Autodesk Fusion 360 part; units mm, degrees
(part 22 of 24)
  line L521 (40.5032, 38.4302) -> (40.7768, 38.4302)
  line L522 (51.1302, 38.2368) -> (51.1302, 37.9632)
  line L523 (50.9368, 37.7698) -> (50.6632, 37.7698)
  line L524 (40.5032, 42.2402) -> (40.7768, 42.2402)
  line L525 (40.7768, 42.2402) -> (40.9702, 42.0468)
  line L526 (50.6632, 42.2402) -> (50.9368, 42.2402)
  line L527 (26.3398, 42.0468) -> (26.5332, 42.2402)
  line L528 (37.1602, 41.7732) -> (36.9668, 41.5798)
  line L529 (50.4698, 38.2368) -> (50.6632, 38.4302)
  line L530 (40.3098, 42.0468) -> (40.5032, 42.2402)
  line L531 (40.9702, 41.7732) -> (40.7768, 41.5798)
  line L532 (51.1302, 42.0468) -> (51.1302, 41.7732)
  line L533 (51.1302, 38.2368) -> (51.1302, 37.9632)
  line L534 (40.5032, 41.5798) -> (40.3098, 41.7732)
  line L535 (50.4698, 41.7732) -> (50.4698, 42.0468)
  line L536 (50.6632, 41.5798) -> (50.4698, 41.7732)
  line L537 (40.7768, 41.5798) -> (40.5032, 41.5798)
  line L538 (50.4698, 41.7732) -> (50.4698, 42.0468)
  line L539 (36.9668, 41.5798) -> (36.6932, 41.5798)
  line L540 (40.3098, 41.7732) -> (40.3098, 42.0468)
  line L541 (26.5332, 41.5798) -> (26.3398, 41.7732)
  line L542 (50.4698, 42.0468) -> (50.6632, 42.2402)
  line L543 (51.1302, 37.9632) -> (50.9368, 37.7698)
  line L544 (50.4698, 41.7732) -> (50.4698, 42.0468)
  line L545 (40.7768, 38.4302) -> (40.9702, 38.2368)
  line L546 (50.4698, 42.0468) -> (50.6632, 42.2402)
  line L547 (50.4698, 41.7732) -> (50.4698, 42.0468)
  line L548 (51.1302, 38.2368) -> (51.1302, 37.9632)
  line L549 (40.9702, 38.2368) -> (40.9702, 37.9632)
  line L550 (40.3098, 41.7732) -> (40.3098, 42.0468)
  line L551 (40.3098, 41.7732) -> (40.3098, 42.0468)
  line L552 (40.5032, 41.5798) -> (40.3098, 41.7732)
  line L553 (50.6632, 41.5798) -> (50.4698, 41.7732)
  line L554 (40.3098, 42.0468) -> (40.5032, 42.2402)
  line L555 (40.3098, 37.9632) -> (40.3098, 38.2368)
  line L556 (50.6632, 42.2402) -> (50.9368, 42.2402)
  line L557 (40.5032, 37.7698) -> (40.3098, 37.9632)
  line L558 (50.9368, 41.5798) -> (50.6632, 41.5798)
  line L559 (40.3098, 38.2368) -> (40.5032, 38.4302)
  line L560 (36.9668, 41.5798) -> (36.6932, 41.5798)
  line L561 (36.4998, 42.0468) -> (36.6932, 42.2402)
  line L562 (4.7498, 15.1032) -> (4.7498, 15.3768)
  line L563 (15.5702, 15.3768) -> (15.5702, 15.1032)
  line L564 (26.8068, 42.2402) -> (27.0002, 42.0468)
  line L565 (5.4102, 15.1032) -> (5.2168, 14.9098)
  line L566 (26.5332, 42.2402) -> (26.8068, 42.2402)
  line L567 (5.2168, 14.9098) -> (4.9432, 14.9098)
  line L568 (26.8068, 42.2402) -> (27.0002, 42.0468)
  line L569 (26.3398, 41.7732) -> (26.3398, 42.0468)
  line L570 (15.3768, 14.9098) -> (15.1032, 14.9098)
  line L571 (15.5702, 15.3768) -> (15.5702, 15.1032)
  line L572 (15.1032, 15.5702) -> (15.3768, 15.5702)
  line L573 (15.3768, 15.5702) -> (15.5702, 15.3768)
  line L574 (26.5332, 42.2402) -> (26.8068, 42.2402)
  line L575 (15.1032, 14.9098) -> (14.9098, 15.1032)
  line L576 (15.3768, 14.9098) -> (15.1032, 14.9098)
  line L577 (4.9432, 15.5702) -> (5.2168, 15.5702)
  line L578 (14.9098, 15.3768) -> (15.1032, 15.5702)
  line L579 (14.9098, 15.3768) -> (15.1032, 15.5702)
  line L580 (15.3768, 15.5702) -> (15.5702, 15.3768)
  line L581 (15.5702, 15.3768) -> (15.5702, 15.1032)
  line L582 (5.4102, 15.3768) -> (5.4102, 15.1032)
  line L583 (5.2168, 14.9098) -> (4.9432, 14.9098)
  line L584 (4.9432, 14.9098) -> (4.7498, 15.1032)
  line L585 (5.2168, 15.5702) -> (5.4102, 15.3768)
  line L586 (5.4102, 15.3768) -> (5.4102, 15.1032)
  line L587 (36.6932, 42.2402) -> (36.9668, 42.2402)
  line L588 (4.7498, 15.3768) -> (4.9432, 15.5702)
  line L589 (27.0002, 41.7732) -> (26.8068, 41.5798)
  line L590 (26.3398, 41.7732) -> (26.3398, 42.0468)
  line L591 (5.4102, 15.3768) -> (5.4102, 15.1032)
  line L592 (4.7498, 15.1032) -> (4.7498, 15.3768)
  line L593 (15.5702, 15.1032) -> (15.3768, 14.9098)
  line L594 (27.0002, 42.0468) -> (27.0002, 41.7732)
  line L595 (36.4998, 42.0468) -> (36.6932, 42.2402)
  line L596 (15.1032, 15.5702) -> (15.3768, 15.5702)
  line L597 (14.9098, 15.1032) -> (14.9098, 15.3768)
  line L598 (37.1602, 42.0468) -> (37.1602, 41.7732)
  line L599 (15.5702, 15.1032) -> (15.3768, 14.9098)
  line L600 (26.3398, 41.7732) -> (26.3398, 42.0468)
  line L601 (26.8068, 41.5798) -> (26.5332, 41.5798)
  line L602 (36.4998, 41.7732) -> (36.4998, 42.0468)
  line L603 (4.7498, 15.3768) -> (4.9432, 15.5702)
  line L604 (5.4102, 15.1032) -> (5.2168, 14.9098)
  line L605 (26.8068, 41.5798) -> (26.5332, 41.5798)
  line L606 (36.4998, 41.7732) -> (36.4998, 42.0468)
  line L607 (27.0002, 41.7732) -> (26.8068, 41.5798)
  line L608 (26.3398, 41.7732) -> (26.3398, 42.0468)
  line L609 (36.6932, 41.5798) -> (36.4998, 41.7732)
  line L610 (36.6932, 42.2402) -> (36.9668, 42.2402)
  line L611 (36.9668, 42.2402) -> (37.1602, 42.0468)
  line L612 (36.6932, 41.5798) -> (36.4998, 41.7732)
  line L613 (27.0002, 42.0468) -> (27.0002, 41.7732)
  line L614 (37.1602, 42.0468) -> (37.1602, 41.7732)
  line L615 (15.5702, 15.3768) -> (15.5702, 15.1032)
  line L616 (14.9098, 15.1032) -> (14.9098, 15.3768)
  line L617 (5.2168, 15.5702) -> (5.4102, 15.3768)
  line L618 (36.9668, 42.2402) -> (37.1602, 42.0468)
  line L619 (37.1602, 41.7732) -> (36.9668, 41.5798)
  line L620 (26.3398, 42.0468) -> (26.5332, 42.2402)
  line L621 (26.5332, 41.5798) -> (26.3398, 41.7732)
  line L622 (15.1032, 14.9098) -> (14.9098, 15.1032)
  line L623 (4.9432, 14.9098) -> (4.7498, 15.1032)
  arc A308 (74.2188, 21.7805) -> (74.2188, 20.8407) centre (74.2188, 21.3106) ccw
  arc A309 (80.7491, 6.9342) -> (80.7491, 7.874) centre (80.7491, 7.4041) ccw
  arc A310 (74.2188, 16.3195) -> (74.2188, 17.2593) centre (74.2188, 16.7894) ccw
  arc A311 (80.7491, 7.874) -> (80.7491, 6.9342) centre (80.7491, 7.4041) ccw
  line L624 (7.8831, 28.575) -> (7.3569, 28.575)
  line L625 (7.8831, 29.845) -> (8.255, 29.4731)
  line L626 (8.255, 29.4731) -> (8.255, 28.9469)
  arc A312 (80.7491, 7.874) -> (80.7491, 6.9342) centre (80.7491, 7.4041) ccw
  arc A313 (80.7212, 17.2593) -> (80.7212, 16.3195) centre (80.7212, 16.7894) ccw
  line L627 (6.985, 28.9469) -> (6.985, 29.4731)
  line L628 (7.3569, 29.845) -> (7.8831, 29.845)
  line L629 (6.985, 21.3269) -> (6.985, 21.8531)
  arc A314 (80.7491, 2.413) -> (80.7491, 3.3528) centre (80.7491, 2.8829) ccw
  line L630 (7.3569, 28.575) -> (6.985, 28.9469)
  arc A315 (80.7212, 16.3195) -> (80.7212, 17.2593) centre (80.7212, 16.7894) ccw
  line L631 (6.985, 28.9469) -> (6.985, 29.4731)
  line L632 (8.255, 21.8531) -> (8.255, 21.3269)
  arc A316 (74.2467, 6.9342) -> (74.2467, 7.874) centre (74.2467, 7.4041) ccw
  arc A317 (80.7212, 20.8407) -> (80.7212, 21.7805) centre (80.7212, 21.3106) ccw
  arc A318 (74.2467, 2.413) -> (74.2467, 3.3528) centre (74.2467, 2.8829) ccw
  arc A319 (74.2188, 20.8407) -> (74.2188, 21.7805) centre (74.2188, 21.3106) ccw
  arc A320 (80.7491, 3.3528) -> (80.7491, 2.413) centre (80.7491, 2.8829) ccw
  arc A321 (80.7212, 20.8407) -> (80.7212, 21.7805) centre (80.7212, 21.3106) ccw
  arc A322 (74.2188, 20.8407) -> (74.2188, 21.7805) centre (74.2188, 21.3106) ccw
  arc A323 (74.2188, 17.2593) -> (74.2188, 16.3195) centre (74.2188, 16.7894) ccw
  arc A324 (74.2188, 17.2593) -> (74.2188, 16.3195) centre (74.2188, 16.7894) ccw
  arc A325 (80.7212, 17.2593) -> (80.7212, 16.3195) centre (80.7212, 16.7894) ccw
  line L633 (4.9432, 15.5702) -> (5.2168, 15.5702)
  arc A326 (74.2467, 7.874) -> (74.2467, 6.9342) centre (74.2467, 7.4041) ccw
  arc A327 (74.2467, 6.9342) -> (74.2467, 7.874) centre (74.2467, 7.4041) ccw
  arc A328 (80.7491, 6.9342) -> (80.7491, 7.874) centre (80.7491, 7.4041) ccw
  arc A329 (80.7212, 21.7805) -> (80.7212, 20.8407) centre (80.7212, 21.3106) ccw
  line L634 (7.8831, 29.845) -> (8.255, 29.4731)
  arc A330 (80.7491, 3.3528) -> (80.7491, 2.413) centre (80.7491, 2.8829) ccw
  arc A331 (80.7212, 21.7805) -> (80.7212, 20.8407) centre (80.7212, 21.3106) ccw
  line L635 (8.255, 29.4731) -> (8.255, 28.9469)
  line L636 (8.255, 28.9469) -> (7.8831, 28.575)
  line L637 (7.8831, 28.575) -> (7.3569, 28.575)
  line L638 (8.255, 28.9469) -> (7.8831, 28.575)
  line L639 (7.3569, 29.845) -> (7.8831, 29.845)
  line L640 (8.255, 21.3269) -> (7.8831, 20.955)
  line L641 (5.4102, 15.3768) -> (5.4102, 15.1032)
  arc A332 (74.2188, 16.3195) -> (74.2188, 17.2593) centre (74.2188, 16.7894) ccw
  line L642 (7.8831, 28.575) -> (7.3569, 28.575)
  line L643 (6.985, 21.8531) -> (7.3569, 22.225)
  arc A333 (80.7491, 2.413) -> (80.7491, 3.3528) centre (80.7491, 2.8829) ccw
  arc A334 (74.2467, 2.413) -> (74.2467, 3.3528) centre (74.2467, 2.8829) ccw
  line L644 (7.8831, 20.955) -> (7.3569, 20.955)
  line L645 (7.8831, 22.225) -> (8.255, 21.8531)
  line L646 (7.8831, 28.575) -> (7.3569, 28.575)
  line L647 (8.255, 21.8531) -> (8.255, 21.3269)
  arc A335 (74.2467, 7.874) -> (74.2467, 6.9342) centre (74.2467, 7.4041) ccw
  line L648 (6.985, 29.4731) -> (7.3569, 29.845)
  line L649 (8.255, 21.3269) -> (7.8831, 20.955)
  line L650 (7.3569, 20.955) -> (6.985, 21.3269)
  line L651 (7.3569, 28.575) -> (6.985, 28.9469)
  arc A336 (74.2467, 3.3528) -> (74.2467, 2.413) centre (74.2467, 2.8829) ccw
  arc A337 (80.7212, 16.3195) -> (80.7212, 17.2593) centre (80.7212, 16.7894) ccw
  arc A338 (74.2188, 21.7805) -> (74.2188, 20.8407) centre (74.2188, 21.3106) ccw
  line L652 (6.985, 29.4731) -> (7.3569, 29.845)
  arc A339 (74.2467, 3.3528) -> (74.2467, 2.413) centre (74.2467, 2.8829) ccw
  line L653 (7.8831, 20.955) -> (7.3569, 20.955)
  line L654 (6.985, 21.3269) -> (6.985, 21.8531)
  line L655 (7.3569, 22.225) -> (7.8831, 22.225)
  arc A340 (20.9804, 37.7698) -> (20.9804, 38.4302) centre (20.9804, 38.1) ccw
  line L656 (7.8831, 20.955) -> (7.3569, 20.955)
  arc A341 (20.9804, 37.7698) -> (20.9804, 38.4302) centre (20.9804, 38.1) ccw
  line L657 (20.9804, 38.1) -> (19.6596, 38.1)
  line L658 (20.9804, 40.64) -> (19.6596, 40.64)
  arc A342 (19.6596, 43.5102) -> (19.6596, 42.8498) centre (19.6596, 43.18) ccw
  line L659 (7.3569, 20.955) -> (6.985, 21.3269)
  arc A343 (20.9804, 40.3098) -> (20.9804, 40.9702) centre (20.9804, 40.64) ccw
  line L660 (20.9804, 43.18) -> (19.6596, 43.18)
  arc A344 (20.9804, 42.8498) -> (20.9804, 43.5102) centre (20.9804, 43.18) ccw
  arc A345 (20.9804, 40.3098) -> (20.9804, 40.9702) centre (20.9804, 40.64) ccw
  line L661 (7.8831, 20.955) -> (7.3569, 20.955)
  arc A346 (19.6596, 43.5102) -> (19.6596, 42.8498) centre (19.6596, 43.18) ccw
  line L662 (20.9804, 38.1) -> (19.6596, 38.1)
  arc A347 (19.6596, 38.4302) -> (19.6596, 37.7698) centre (19.6596, 38.1) ccw
  arc A348 (19.6596, 38.4302) -> (19.6596, 37.7698) centre (19.6596, 38.1) ccw
  line L663 (7.8831, 22.225) -> (8.255, 21.8531)
  arc A349 (19.6596, 40.9702) -> (19.6596, 40.3098) centre (19.6596, 40.64) ccw
  arc A350 (19.6596, 40.9702) -> (19.6596, 40.3098) centre (19.6596, 40.64) ccw
  line L664 (7.3569, 22.225) -> (7.8831, 22.225)
  line L665 (6.985, 21.8531) -> (7.3569, 22.225)
  line L666 (20.9804, 40.64) -> (19.6596, 40.64)
  arc A351 (20.9804, 42.8498) -> (20.9804, 43.5102) centre (20.9804, 43.18) ccw
  line L667 (20.9804, 43.18) -> (19.6596, 43.18)
  line L668 (10.9601, 50.4698) -> (10.9601, 48.5902)
  line L669 (11.8999, 48.5902) -> (11.8999, 50.4698)
  line L670 (13.5001, 50.4698) -> (13.5001, 48.5902)
  line L671 (14.4399, 48.5902) -> (14.4399, 50.4698)
  line L672 (16.0401, 50.4698) -> (16.0401, 48.5902)
  line L673 (16.9799, 50.4698) -> (16.9799, 48.5902)
  line L674 (18.5801, 48.5902) -> (18.5801, 50.4698)
  line L675 (19.5199, 50.4698) -> (19.5199, 48.5902)
  line L676 (21.1201, 48.5902) -> (21.1201, 50.4698)
  line L677 (22.0599, 50.4698) -> (22.0599, 48.5902)
  line L678 (20.9804, 43.5102) -> (19.6596, 43.5102)
  line L679 (19.6596, 42.8498) -> (20.9804, 42.8498)
  line L680 (20.9804, 40.9702) -> (19.6596, 40.9702)
  line L681 (19.6596, 40.3098) -> (20.9804, 40.3098)
  line L682 (20.9804, 38.4302) -> (19.6596, 38.4302)
  line L683 (19.6596, 37.7698) -> (20.9804, 37.7698)
  line L684 (3.7084, 44.7802) -> (2.3876, 44.7802)
  line L685 (2.3876, 44.1198) -> (3.7084, 44.1198)
  line L686 (7.4676, 44.7802) -> (8.7884, 44.7802)
  line L687 (8.7884, 44.1198) -> (7.4676, 44.1198)
  line L688 (7.4676, 42.2402) -> (8.7884, 42.2402)
  line L689 (8.7884, 41.5798) -> (7.4676, 41.5798)
  line L690 (3.7084, 42.2402) -> (2.3876, 42.2402)
  line L691 (2.3876, 41.5798) -> (3.7084, 41.5798)
  line L692 (2.3876, 34.6202) -> (3.7084, 34.6202)
  line L693 (3.7084, 33.9598) -> (2.3876, 33.9598)
  line L694 (8.7884, 34.6202) -> (7.4676, 34.6202)
  line L695 (7.4676, 33.9598) -> (8.7884, 33.9598)
  line L696 (26.2001, 26.3398) -> (26.2001, 24.4602)
  line L697 (27.1399, 26.3398) -> (27.1399, 24.4602)
  line L698 (28.7401, 26.3398) -> (28.7401, 24.4602)
  line L699 (29.6799, 26.3398) -> (29.6799, 24.4602)
  line L700 (31.2801, 24.4602) -> (31.2801, 26.3398)
  line L701 (32.2199, 26.3398) -> (32.2199, 24.4602)
  line L702 (33.8201, 24.4602) -> (33.8201, 26.3398)
  line L703 (34.7599, 26.3398) -> (34.7599, 24.4602)
  line L704 (36.3601, 24.4602) -> (36.3601, 26.3398)
  line L705 (37.2999, 26.3398) -> (37.2999, 24.4602)
  line L706 (47.7901, 26.3398) -> (47.7901, 24.4602)
  line L707 (48.7299, 24.4602) -> (48.7299, 26.3398)
  line L708 (50.3301, 26.3398) -> (50.3301, 24.4602)
  line L709 (51.2699, 24.4602) -> (51.2699, 26.3398)
  line L710 (52.8701, 26.3398) -> (52.8701, 24.4602)
  line L711 (53.8099, 24.4602) -> (53.8099, 26.3398)
  line L712 (60.4901, 30.8102) -> (60.4901, 32.6898)
  line L713 (61.4299, 30.8102) -> (61.4299, 32.6898)
  line L714 (63.0301, 32.6898) -> (63.0301, 30.8102)
  line L715 (63.9699, 30.8102) -> (63.9699, 32.6898)
  line L716 (65.5701, 32.6898) -> (65.5701, 30.8102)
  line L717 (66.5099, 30.8102) -> (66.5099, 32.6898)
  line L718 (73.1901, 32.6898) -> (73.1901, 30.8102)
  line L719 (74.1299, 30.8102) -> (74.1299, 32.6898)
  line L720 (75.7301, 32.6898) -> (75.7301, 30.8102)
  line L721 (76.6699, 30.8102) -> (76.6699, 32.6898)
  line L722 (78.2701, 32.6898) -> (78.2701, 30.8102)
  line L723 (79.2099, 30.8102) -> (79.2099, 32.6898)
  line L724 (80.8101, 32.6898) -> (80.8101, 30.8102)
  line L725 (81.7499, 30.8102) -> (81.7499, 32.6898)
  line L726 (57.9501, 44.1198) -> (57.9501, 42.2402)
  line L727 (58.8899, 42.2402) -> (58.8899, 44.1198)
  line L728 (60.4901, 44.1198) -> (60.4901, 42.2402)
  line L729 (61.4299, 42.2402) -> (61.4299, 44.1198)
  line L730 (63.0301, 44.1198) -> (63.0301, 42.2402)
  line L731 (63.9699, 42.2402) -> (63.9699, 44.1198)
  line L732 (65.5701, 44.1198) -> (65.5701, 42.2402)
  line L733 (66.5099, 42.2402) -> (66.5099, 44.1198)
  line L734 (73.1901, 45.3898) -> (73.1901, 43.5102)
  line L735 (74.1299, 43.5102) -> (74.1299, 45.3898)
  line L736 (75.7301, 45.3898) -> (75.7301, 43.5102)
  line L737 (76.6699, 43.5102) -> (76.6699, 45.3898)
  line L738 (79.2099, 45.3898) -> (79.2099, 43.5102)
  line L739 (78.2701, 43.5102) -> (78.2701, 45.3898)
  line L740 (80.8101, 45.3898) -> (80.8101, 43.5102)
  line L741 (81.7499, 43.5102) -> (81.7499, 45.3898)
  constraint tangent A238 L668
  constraint tangent A222 L669
  constraint tangent A226 L670
  constraint tangent A221 L671
  constraint tangent A236 L672
  constraint tangent A231 L673
  constraint tangent A217 L674
  constraint tangent A225 L675
  constraint tangent A224 L676
  constraint tangent A237 L677
  constraint tangent A346 L678
  constraint tangent A344 L679
  constraint tangent A349 L680
  constraint tangent A350 L681
  constraint parallel L680 L681
  constraint tangent A347 L682
  constraint tangent A341 L683
  constraint tangent A280 L684
  constraint tangent A283 L685
  constraint tangent A292 L686
  constraint tangent A297 L687
  constraint tangent A295 L688
  constraint tangent A289 L689
  constraint tangent A296 L690
  constraint tangent A288 L691
  constraint tangent A303 L692
  constraint tangent A301 L693
  constraint tangent A293 L694
  constraint tangent A286 L695
  constraint tangent A153 L696
  constraint tangent A100 L697
  constraint tangent A136 L698
  constraint tangent A136 L699
  constraint tangent A151 L700
  constraint tangent A154 L701
  constraint tangent A152 L702
  constraint tangent A152 L703
  constraint tangent A149 L704
  constraint tangent A147 L705
  constraint tangent A252 L706
  constraint tangent A264 L707
  constraint tangent A257 L708
  constraint tangent A249 L709
  constraint tangent A268 L710
  constraint tangent A266 L711
  constraint tangent A213 L712
  constraint tangent A213 L713
  constraint tangent A198 L714
  constraint tangent A229 L715
  constraint tangent A218 L716
  constraint tangent A218 L717
  constraint tangent A163 L718
  constraint tangent A180 L719
  constraint tangent A168 L720
  constraint tangent A170 L721
  constraint tangent A208 L722
  constraint tangent A208 L723
  constraint tangent A206 L724
  constraint tangent A186 L725
  constraint tangent A209 L726
  constraint tangent A209 L727
  constraint tangent A187 L728
  constraint tangent A204 L729
  constraint tangent A195 L730
  constraint tangent A194 L731
  constraint tangent A185 L732
  constraint tangent A191 L733
  constraint tangent A160 L734
  constraint tangent A169 L735
  constraint tangent A176 L736
  constraint tangent A166 L737
  constraint tangent A181 L738
  constraint tangent A159 L739
  constraint tangent A162 L740
  constraint tangent A158 L741
sketch "Bottom Component Outlines" plane through (0, 0, 0) normal (0, 0, 1) x (1, 0, 0)
  arc A0 (46.3191, 48.2959) -> (46.3909, 48.2241) centre (46.355, 48.26) ccw
  line L0 (59.055, 7.62) -> (57.785, 7.62)
  arc A1 (67.9809, 7.5841) -> (67.9091, 7.6559) centre (67.945, 7.62) ccw
  arc A2 (67.2741, 7.0209) -> (67.3459, 6.9491) centre (67.31, 6.985) ccw
  arc A3 (52.705, 7.6708) -> (52.705, 7.5692) centre (52.705, 7.62) ccw
  arc A4 (53.9391, 5.1159) -> (54.0109, 5.0441) centre (53.975, 5.08) ccw
  arc A5 (51.3991, 5.1159) -> (51.4709, 5.0441) centre (51.435, 5.08) ccw
  arc A6 (49.4941, 7.0209) -> (49.5659, 6.9491) centre (49.53, 6.985) ccw
  arc A7 (69.215, 7.5692) -> (69.215, 7.6708) centre (69.215, 7.62) ccw
  arc A8 (49.5659, 5.7509) -> (49.4941, 5.6791) centre (49.53, 5.715) ccw
  arc A9 (52.705, 5.1308) -> (52.705, 5.0292) centre (52.705, 5.08) ccw
  arc A10 (67.9091, 5.0441) -> (67.9809, 5.1159) centre (67.945, 5.08) ccw
  arc A11 (54.5741, 6.9491) -> (54.6459, 7.0209) centre (54.61, 6.985) ccw
  line L1 (52.07, 6.985) -> (51.435, 7.62)
  line L2 (54.61, 6.985) -> (53.975, 7.62)
  line L3 (52.07, 5.715) -> (52.705, 5.08)
  line L4 (51.435, 5.08) -> (52.07, 5.715)
  arc A12 (52.7409, 7.5841) -> (52.6691, 7.6559) centre (52.705, 7.62) ccw
  arc A13 (50.1291, 5.0441) -> (50.2009, 5.1159) centre (50.165, 5.08) ccw
  arc A14 (54.6459, 5.6791) -> (54.5741, 5.7509) centre (54.61, 5.715) ccw
  arc A15 (69.7992, 5.715) -> (69.9008, 5.715) centre (69.85, 5.715) ccw
  arc A16 (51.4709, 7.6559) -> (51.3991, 7.5841) centre (51.435, 7.62) ccw
  arc A17 (46.3909, 50.8359) -> (46.3191, 50.7641) centre (46.355, 50.8) ccw
  line L5 (69.85, 6.985) -> (69.215, 7.62)
  arc A18 (52.1059, 5.7509) -> (52.0341, 5.6791) centre (52.07, 5.715) ccw
  line L6 (69.85, 5.715) -> (69.85, 6.985)
  arc A19 (69.1791, 5.1159) -> (69.2509, 5.0441) centre (69.215, 5.08) ccw
  arc A20 (54.0109, 7.6559) -> (53.9391, 7.5841) centre (53.975, 7.62) ccw
  line L7 (52.705, 5.08) -> (53.975, 5.08)
  arc A21 (52.0341, 7.0209) -> (52.1059, 6.9491) centre (52.07, 6.985) ccw
  arc A22 (69.2509, 7.6559) -> (69.1791, 7.5841) centre (69.215, 7.62) ccw
  line L8 (45.085, 48.26) -> (46.355, 48.26)
  arc A23 (52.705, 50.8508) -> (52.705, 50.7492) centre (52.705, 50.8) ccw
  arc A24 (69.9008, 6.985) -> (69.7992, 6.985) centre (69.85, 6.985) ccw
  line L9 (67.31, 6.985) -> (67.945, 7.62)
  arc A25 (53.975, 7.5692) -> (53.975, 7.6708) centre (53.975, 7.62) ccw
  line L10 (52.705, 7.62) -> (52.07, 6.985)
  arc A26 (52.1059, 5.6791) -> (52.0341, 5.7509) centre (52.07, 5.715) ccw
  arc A27 (52.6691, 5.0441) -> (52.7409, 5.1159) centre (52.705, 5.08) ccw
  line L11 (53.975, 7.62) -> (52.705, 7.62)
  arc A28 (51.435, 7.5692) -> (51.435, 7.6708) centre (51.435, 7.62) ccw
  arc A29 (67.945, 5.1308) -> (67.945, 5.0292) centre (67.945, 5.08) ccw
  line L12 (69.215, 5.08) -> (69.85, 5.715)
  arc A30 (50.165, 5.1308) -> (50.165, 5.0292) centre (50.165, 5.08) ccw
  arc A31 (57.785, 7.6708) -> (57.785, 7.5692) centre (57.785, 7.62) ccw
  arc A32 (47.0259, 48.8591) -> (46.9541, 48.9309) centre (46.99, 48.895) ccw
  arc A33 (59.055, 7.5692) -> (59.055, 7.6708) centre (59.055, 7.62) ccw
  arc A34 (69.215, 5.0292) -> (69.215, 5.1308) centre (69.215, 5.08) ccw
  arc A35 (51.435, 5.0292) -> (51.435, 5.1308) centre (51.435, 5.08) ccw
  line L13 (53.975, 5.08) -> (54.61, 5.715)
  line L14 (51.435, 7.62) -> (50.165, 7.62)
  line L15 (50.165, 5.08) -> (49.53, 5.715)
  line L16 (69.215, 7.62) -> (67.945, 7.62)
  arc A36 (67.945, 7.6708) -> (67.945, 7.5692) centre (67.945, 7.62) ccw
  line L17 (67.945, 5.08) -> (67.31, 5.715)
  arc A37 (50.2009, 7.5841) -> (50.1291, 7.6559) centre (50.165, 7.62) ccw
  arc A38 (50.165, 7.6708) -> (50.165, 7.5692) centre (50.165, 7.62) ccw
  line L18 (52.07, 48.895) -> (52.705, 48.26)
  arc A39 (52.0341, 6.9491) -> (52.1059, 7.0209) centre (52.07, 6.985) ccw
  line L19 (67.945, 5.08) -> (69.215, 5.08)
  line L20 (50.165, 5.08) -> (51.435, 5.08)
  line L21 (49.53, 6.985) -> (50.165, 7.62)
  arc A40 (67.3459, 5.7509) -> (67.2741, 5.6791) centre (67.31, 5.715) ccw
  arc A41 (69.8859, 5.6791) -> (69.8141, 5.7509) centre (69.85, 5.715) ccw
  arc A42 (52.0341, 50.2009) -> (52.1059, 50.1291) centre (52.07, 50.165) ccw
  arc A43 (46.9541, 50.2009) -> (47.0259, 50.1291) centre (46.99, 50.165) ccw
  line L22 (53.975, 50.8) -> (52.705, 50.8)
  arc A44 (46.355, 48.2092) -> (46.355, 48.3108) centre (46.355, 48.26) ccw
  arc A45 (45.0491, 48.2241) -> (45.1209, 48.2959) centre (45.085, 48.26) ccw
  arc A46 (48.895, 50.7492) -> (48.895, 50.8508) centre (48.895, 50.8) ccw
  arc A47 (45.085, 48.3108) -> (45.085, 48.2092) centre (45.085, 48.26) ccw
  line L23 (48.895, 50.8) -> (47.625, 50.8)
  line L24 (46.355, 50.8) -> (45.085, 50.8)
  line L25 (47.625, 50.8) -> (46.99, 50.165)
  arc A48 (49.4941, 50.1291) -> (49.5659, 50.2009) centre (49.53, 50.165) ccw
  line L26 (44.45, 48.895) -> (45.085, 48.26)
  arc A49 (49.5659, 48.8591) -> (49.4941, 48.9309) centre (49.53, 48.895) ccw
  arc A50 (46.9541, 50.1291) -> (47.0259, 50.2009) centre (46.99, 50.165) ccw
  arc A51 (44.4859, 48.9309) -> (44.4141, 48.8591) centre (44.45, 48.895) ccw
  arc A52 (45.1209, 50.7641) -> (45.0491, 50.8359) centre (45.085, 50.8) ccw
  arc A53 (50.2009, 50.7641) -> (50.1291, 50.8359) centre (50.165, 50.8) ccw
  arc A54 (44.4141, 50.2009) -> (44.4859, 50.1291) centre (44.45, 50.165) ccw
  line L27 (49.53, 50.165) -> (48.895, 50.8)
  line L28 (47.625, 48.26) -> (48.895, 48.26)
  line L29 (55.245, 48.26) -> (56.515, 48.26)
  arc A55 (47.0259, 48.9309) -> (46.9541, 48.8591) centre (46.99, 48.895) ccw
  line L30 (52.07, 50.165) -> (51.435, 50.8)
  line L31 (45.085, 50.8) -> (44.45, 50.165)
  arc A56 (52.7409, 50.7641) -> (52.6691, 50.8359) centre (52.705, 50.8) ccw
  arc A57 (47.6609, 50.7641) -> (47.5891, 50.8359) centre (47.625, 50.8) ccw
  arc A58 (46.355, 50.7492) -> (46.355, 50.8508) centre (46.355, 50.8) ccw
  line L32 (49.53, 48.895) -> (50.165, 48.26)
  arc A59 (55.2091, 48.2241) -> (55.2809, 48.2959) centre (55.245, 48.26) ccw
  arc A60 (47.5891, 48.2241) -> (47.6609, 48.2959) centre (47.625, 48.26) ccw
  line L33 (46.99, 48.895) -> (46.355, 48.26)
  line L34 (56.515, 50.8) -> (55.245, 50.8)
  arc A61 (53.975, 48.2092) -> (53.975, 48.3108) centre (53.975, 48.26) ccw
  arc A62 (48.8591, 48.2959) -> (48.9309, 48.2241) centre (48.895, 48.26) ccw
  arc A63 (48.895, 48.2092) -> (48.895, 48.3108) centre (48.895, 48.26) ccw
  line L35 (52.705, 50.8) -> (52.07, 50.165)
  arc A64 (47.625, 50.8508) -> (47.625, 50.7492) centre (47.625, 50.8) ccw
  arc A65 (48.9309, 50.8359) -> (48.8591, 50.7641) centre (48.895, 50.8) ccw
  arc A66 (53.975, 50.7492) -> (53.975, 50.8508) centre (53.975, 50.8) ccw
  arc A67 (45.085, 50.8508) -> (45.085, 50.7492) centre (45.085, 50.8) ccw
  arc A68 (47.625, 48.3108) -> (47.625, 48.2092) centre (47.625, 48.26) ccw
  line L36 (46.99, 48.895) -> (47.625, 48.26)
  line L37 (48.895, 48.26) -> (49.53, 48.895)
  line L38 (46.355, 50.8) -> (46.99, 50.165)
  arc A69 (59.055, 50.7492) -> (59.055, 50.8508) centre (59.055, 50.8) ccw
  arc A70 (51.435, 50.7492) -> (51.435, 50.8508) centre (51.435, 50.8) ccw
  arc A71 (50.165, 50.8508) -> (50.165, 50.7492) centre (50.165, 50.8) ccw
  arc A72 (56.515, 50.7492) -> (56.515, 50.8508) centre (56.515, 50.8) ccw
  line L39 (59.055, 50.8) -> (57.785, 50.8)
  line L40 (50.165, 50.8) -> (49.53, 50.165)
  arc A73 (59.6541, 50.1291) -> (59.7259, 50.2009) centre (59.69, 50.165) ccw
  arc A74 (61.595, 50.7492) -> (61.595, 50.8508) centre (61.595, 50.8) ccw
  arc A75 (52.1059, 48.9309) -> (52.0341, 48.8591) centre (52.07, 48.895) ccw
  line L41 (54.61, 48.895) -> (55.245, 48.26)
  arc A76 (54.6459, 48.8591) -> (54.5741, 48.9309) centre (54.61, 48.895) ccw
  arc A77 (55.245, 50.8508) -> (55.245, 50.7492) centre (55.245, 50.8) ccw
  arc A78 (60.2891, 48.2241) -> (60.3609, 48.2959) centre (60.325, 48.26) ccw
  arc A79 (52.6691, 48.2241) -> (52.7409, 48.2959) centre (52.705, 48.26) ccw
  arc A80 (60.3609, 50.7641) -> (60.2891, 50.8359) centre (60.325, 50.8) ccw
  arc A81 (52.0341, 50.1291) -> (52.1059, 50.2009) centre (52.07, 50.165) ccw
  arc A82 (51.4709, 50.8359) -> (51.3991, 50.7641) centre (51.435, 50.8) ccw
  line L42 (61.595, 50.8) -> (60.325, 50.8)
  line L43 (51.435, 50.8) -> (50.165, 50.8)
  arc A83 (57.1141, 50.1291) -> (57.1859, 50.2009) centre (57.15, 50.165) ccw
  line L44 (57.15, 50.165) -> (56.515, 50.8)
  arc A84 (50.165, 48.3108) -> (50.165, 48.2092) centre (50.165, 48.26) ccw
  arc A85 (55.2809, 50.7641) -> (55.2091, 50.8359) centre (55.245, 50.8) ccw
  line L45 (51.435, 48.26) -> (52.07, 48.895)
  arc A86 (57.1141, 50.2009) -> (57.1859, 50.1291) centre (57.15, 50.165) ccw
  arc A87 (51.435, 48.2092) -> (51.435, 48.3108) centre (51.435, 48.26) ccw
  arc A88 (55.245, 48.3108) -> (55.245, 48.2092) centre (55.245, 48.26) ccw
  arc A89 (52.705, 48.3108) -> (52.705, 48.2092) centre (52.705, 48.26) ccw
  arc A90 (60.325, 50.8508) -> (60.325, 50.7492) centre (60.325, 50.8) ccw
  line L46 (59.69, 48.895) -> (60.325, 48.26)
  arc A91 (49.5659, 48.9309) -> (49.4941, 48.8591) centre (49.53, 48.895) ccw
  line L47 (54.61, 48.895) -> (53.975, 48.26)
  line L48 (50.165, 48.26) -> (51.435, 48.26)
  line L49 (57.785, 50.8) -> (57.15, 50.165)
  arc A92 (56.5509, 50.8359) -> (56.4791, 50.7641) centre (56.515, 50.8) ccw
  arc A93 (54.5741, 50.1291) -> (54.6459, 50.2009) centre (54.61, 50.165) ccw
  arc A94 (49.4941, 50.2009) -> (49.5659, 50.1291) centre (49.53, 50.165) ccw
  arc A95 (53.9391, 48.2959) -> (54.0109, 48.2241) centre (53.975, 48.26) ccw
  arc A96 (52.1059, 48.8591) -> (52.0341, 48.9309) centre (52.07, 48.895) ccw
  line L50 (52.705, 48.26) -> (53.975, 48.26)
  arc A97 (54.6459, 48.9309) -> (54.5741, 48.8591) centre (54.61, 48.895) ccw
  arc A98 (54.5741, 50.2009) -> (54.6459, 50.1291) centre (54.61, 50.165) ccw
  arc A99 (57.785, 50.8508) -> (57.785, 50.7492) centre (57.785, 50.8) ccw
  arc A100 (57.1859, 48.8591) -> (57.1141, 48.9309) centre (57.15, 48.895) ccw
  arc A101 (59.0191, 48.2959) -> (59.0909, 48.2241) centre (59.055, 48.26) ccw
  arc A102 (51.3991, 48.2959) -> (51.4709, 48.2241) centre (51.435, 48.26) ccw
  line L51 (57.785, 48.26) -> (59.055, 48.26)
  line L52 (60.325, 50.8) -> (59.69, 50.165)
  arc A103 (54.0109, 50.8359) -> (53.9391, 50.7641) centre (53.975, 50.8) ccw
  line L53 (56.515, 48.26) -> (57.15, 48.895)
  line L54 (59.69, 50.165) -> (59.055, 50.8)
  arc A104 (59.0909, 50.8359) -> (59.0191, 50.7641) centre (59.055, 50.8) ccw
  line L55 (55.245, 50.8) -> (54.61, 50.165)
  arc A105 (28.575, 50.7492) -> (28.575, 50.8508) centre (28.575, 50.8) ccw
  arc A106 (26.7059, 48.9309) -> (26.6341, 48.8591) centre (26.67, 48.895) ccw
  arc A107 (29.2459, 48.9309) -> (29.1741, 48.8591) centre (29.21, 48.895) ccw
  arc A108 (26.6341, 50.2009) -> (26.7059, 50.1291) centre (26.67, 50.165) ccw
  arc A109 (31.1509, 50.8359) -> (31.0791, 50.7641) centre (31.115, 50.8) ccw
  line L56 (34.925, 50.8) -> (34.29, 50.165)
  arc A110 (56.4791, 48.2959) -> (56.5509, 48.2241) centre (56.515, 48.26) ccw
  line L57 (28.575, 50.8) -> (29.21, 50.165)
  arc A111 (56.515, 48.2092) -> (56.515, 48.3108) centre (56.515, 48.26) ccw
  arc A112 (57.785, 48.3108) -> (57.785, 48.2092) centre (57.785, 48.26) ccw
  arc A113 (62.2659, 48.8591) -> (62.1941, 48.9309) centre (62.23, 48.895) ccw
  line L58 (29.21, 48.895) -> (28.575, 48.26)
  arc A114 (29.1741, 50.2009) -> (29.2459, 50.1291) centre (29.21, 50.165) ccw
  line L59 (59.055, 48.26) -> (59.69, 48.895)
  line L60 (29.845, 48.26) -> (31.115, 48.26)
  arc A115 (50.1291, 48.2241) -> (50.2009, 48.2959) centre (50.165, 48.26) ccw
  arc A116 (62.1941, 50.1291) -> (62.2659, 50.2009) centre (62.23, 50.165) ccw
  arc A117 (62.1792, 48.895) -> (62.2808, 48.895) centre (62.23, 48.895) ccw
  arc A118 (34.9609, 50.7641) -> (34.8891, 50.8359) centre (34.925, 50.8) ccw
  arc A119 (31.115, 48.2092) -> (31.115, 48.3108) centre (31.115, 48.26) ccw
  line L61 (29.845, 50.8) -> (29.21, 50.165)
  line L62 (31.75, 50.165) -> (31.115, 50.8)
  line L63 (27.305, 50.8) -> (26.67, 50.165)
  arc A120 (59.6541, 50.2009) -> (59.7259, 50.1291) centre (59.69, 50.165) ccw
  arc A121 (27.3409, 50.7641) -> (27.2691, 50.8359) centre (27.305, 50.8) ccw
  arc A122 (57.7491, 48.2241) -> (57.8209, 48.2959) centre (57.785, 48.26) ccw
  arc A123 (34.2541, 50.2009) -> (34.3259, 50.1291) centre (34.29, 50.165) ccw
  arc A124 (61.595, 48.2092) -> (61.595, 48.3108) centre (61.595, 48.26) ccw
  arc A125 (31.115, 50.7492) -> (31.115, 50.8508) centre (31.115, 50.8) ccw
  line L64 (53.975, 50.8) -> (54.61, 50.165)
  arc A126 (62.2808, 50.165) -> (62.1792, 50.165) centre (62.23, 50.165) ccw
  arc A127 (59.7259, 48.9309) -> (59.6541, 48.8591) centre (59.69, 48.895) ccw
  arc A128 (34.925, 50.8508) -> (34.925, 50.7492) centre (34.925, 50.8) ccw
  line L65 (62.23, 50.165) -> (62.23, 48.895)
  line L66 (62.23, 48.895) -> (61.595, 48.26)
  arc A129 (59.7259, 48.8591) -> (59.6541, 48.9309) centre (59.69, 48.895) ccw
  arc A130 (36.8659, 48.8591) -> (36.7941, 48.9309) centre (36.83, 48.895) ccw
  arc A131 (37.465, 48.3108) -> (37.465, 48.2092) centre (37.465, 48.26) ccw
  arc A132 (36.8659, 48.9309) -> (36.7941, 48.8591) centre (36.83, 48.895) ccw
  arc A133 (39.4059, 48.8591) -> (39.3341, 48.9309) centre (39.37, 48.895) ccw
  line L67 (57.15, 48.895) -> (57.785, 48.26)
  arc A134 (60.325, 48.3108) -> (60.325, 48.2092) centre (60.325, 48.26) ccw
  arc A135 (29.8809, 50.7641) -> (29.8091, 50.8359) centre (29.845, 50.8) ccw
  arc A136 (29.2459, 48.8591) -> (29.1741, 48.9309) centre (29.21, 48.895) ccw
  line L68 (60.325, 48.26) -> (61.595, 48.26)
  line L69 (29.21, 48.895) -> (29.845, 48.26)
  line L70 (31.115, 48.26) -> (31.75, 48.895)
  arc A137 (29.845, 50.8508) -> (29.845, 50.7492) centre (29.845, 50.8) ccw
  arc A138 (61.5591, 48.2959) -> (61.6309, 48.2241) centre (61.595, 48.26) ccw
  arc A139 (34.3259, 48.8591) -> (34.2541, 48.9309) centre (34.29, 48.895) ccw
  line L71 (34.29, 50.165) -> (33.655, 50.8)
  arc A140 (43.815, 50.7492) -> (43.815, 50.8508) centre (43.815, 50.8) ccw
  arc A141 (57.8209, 50.7641) -> (57.7491, 50.8359) centre (57.785, 50.8) ccw
  line L72 (32.385, 50.8) -> (31.75, 50.165)
  arc A142 (61.6309, 50.8359) -> (61.5591, 50.7641) centre (61.595, 50.8) ccw
  line L73 (27.305, 48.26) -> (28.575, 48.26)
  arc A143 (27.305, 50.8508) -> (27.305, 50.7492) centre (27.305, 50.8) ccw
  line L74 (36.195, 50.8) -> (36.83, 50.165)
  line L75 (31.115, 50.8) -> (29.845, 50.8)
  arc A144 (28.5391, 48.2959) -> (28.6109, 48.2241) centre (28.575, 48.26) ccw
  arc A145 (31.7141, 50.1291) -> (31.7859, 50.2009) centre (31.75, 50.165) ccw
  arc A146 (29.8091, 48.2241) -> (29.8809, 48.2959) centre (29.845, 48.26) ccw
  line L76 (26.67, 48.895) -> (27.305, 48.26)
  arc A147 (57.1859, 48.9309) -> (57.1141, 48.8591) centre (57.15, 48.895) ccw
  arc A148 (31.7859, 48.8591) -> (31.7141, 48.9309) centre (31.75, 48.895) ccw
  arc A149 (34.2541, 50.1291) -> (34.3259, 50.2009) centre (34.29, 50.165) ccw
  line L77 (28.575, 50.8) -> (27.305, 50.8)
  line L78 (36.195, 50.8) -> (34.925, 50.8)
  arc A150 (29.1741, 50.1291) -> (29.2459, 50.2009) centre (29.21, 50.165) ccw
  arc A151 (31.0791, 48.2959) -> (31.1509, 48.2241) centre (31.115, 48.26) ccw
  arc A152 (27.2691, 48.2241) -> (27.3409, 48.2959) centre (27.305, 48.26) ccw
  arc A153 (36.195, 50.7492) -> (36.195, 50.8508) centre (36.195, 50.8) ccw
  line L79 (36.83, 48.895) -> (37.465, 48.26)
  arc A154 (28.6109, 50.8359) -> (28.5391, 50.7641) centre (28.575, 50.8) ccw
  line L80 (33.655, 50.8) -> (32.385, 50.8)
  arc A155 (41.9459, 48.9309) -> (41.8741, 48.8591) centre (41.91, 48.895) ccw
  arc A156 (29.845, 48.3108) -> (29.845, 48.2092) centre (29.845, 48.26) ccw
  arc A157 (59.055, 48.2092) -> (59.055, 48.3108) centre (59.055, 48.26) ccw
  line L81 (61.595, 50.8) -> (62.23, 50.165)
  arc A158 (28.575, 48.2092) -> (28.575, 48.3108) centre (28.575, 48.26) ccw
  arc A159 (27.305, 48.3108) -> (27.305, 48.2092) centre (27.305, 48.26) ccw
  arc A160 (32.385, 48.3108) -> (32.385, 48.2092) centre (32.385, 48.26) ccw
  line L82 (34.29, 48.895) -> (34.925, 48.26)
  arc A161 (42.5809, 50.7641) -> (42.5091, 50.8359) centre (42.545, 50.8) ccw
  line L83 (31.75, 48.895) -> (32.385, 48.26)
  arc A162 (42.545, 50.8508) -> (42.545, 50.7492) centre (42.545, 50.8) ccw
  line L84 (32.385, 48.26) -> (33.655, 48.26)
  line L85 (33.655, 48.26) -> (34.29, 48.895)
  arc A163 (39.3341, 50.1291) -> (39.4059, 50.2009) centre (39.37, 50.165) ccw
  line L86 (41.91, 48.895) -> (42.545, 48.26)
  arc A164 (33.655, 50.7492) -> (33.655, 50.8508) centre (33.655, 50.8) ccw
  arc A165 (42.5091, 48.2241) -> (42.5809, 48.2959) centre (42.545, 48.26) ccw
  arc A166 (41.3109, 50.8359) -> (41.2391, 50.7641) centre (41.275, 50.8) ccw
  line L87 (43.815, 50.8) -> (42.545, 50.8)
  arc A167 (36.2309, 50.8359) -> (36.1591, 50.7641) centre (36.195, 50.8) ccw
  arc A168 (34.8891, 48.2241) -> (34.9609, 48.2959) centre (34.925, 48.26) ccw
  arc A169 (38.7709, 50.8359) -> (38.6991, 50.7641) centre (38.735, 50.8) ccw
  line L88 (38.735, 48.26) -> (39.37, 48.895)
  arc A170 (36.1591, 48.2959) -> (36.2309, 48.2241) centre (36.195, 48.26) ccw
  line L89 (41.91, 50.165) -> (41.275, 50.8)
  arc A171 (32.3491, 48.2241) -> (32.4209, 48.2959) centre (32.385, 48.26) ccw
  arc A172 (33.6909, 50.8359) -> (33.6191, 50.7641) centre (33.655, 50.8) ccw
  line L90 (40.005, 50.8) -> (39.37, 50.165)
  line L91 (36.83, 48.895) -> (36.195, 48.26)
  line L92 (42.545, 50.8) -> (41.91, 50.165)
  arc A173 (33.655, 48.2092) -> (33.655, 48.3108) centre (33.655, 48.26) ccw
  arc A174 (33.6191, 48.2959) -> (33.6909, 48.2241) centre (33.655, 48.26) ccw
  arc A175 (32.4209, 50.7641) -> (32.3491, 50.8359) centre (32.385, 50.8) ccw
  line L93 (37.465, 50.8) -> (36.83, 50.165)
  arc A176 (31.7859, 48.9309) -> (31.7141, 48.8591) centre (31.75, 48.895) ccw
  line L94 (34.925, 48.26) -> (36.195, 48.26)
  arc A177 (36.195, 48.2092) -> (36.195, 48.3108) centre (36.195, 48.26) ccw
  arc A178 (36.7941, 50.1291) -> (36.8659, 50.2009) centre (36.83, 50.165) ccw
  line L95 (38.735, 50.8) -> (37.465, 50.8)
  arc A179 (34.925, 48.3108) -> (34.925, 48.2092) centre (34.925, 48.26) ccw
  arc A180 (37.5009, 50.7641) -> (37.4291, 50.8359) centre (37.465, 50.8) ccw
  arc A181 (31.7141, 50.2009) -> (31.7859, 50.1291) centre (31.75, 50.165) ccw
  arc A182 (38.735, 48.2092) -> (38.735, 48.3108) centre (38.735, 48.26) ccw
  arc A183 (40.005, 50.8508) -> (40.005, 50.7492) centre (40.005, 50.8) ccw
  arc A184 (37.465, 50.8508) -> (37.465, 50.7492) centre (37.465, 50.8) ccw
  arc A185 (41.8741, 50.2009) -> (41.9459, 50.1291) centre (41.91, 50.165) ccw
  line L96 (37.465, 48.26) -> (38.735, 48.26)
  arc A186 (38.6991, 48.2959) -> (38.7709, 48.2241) centre (38.735, 48.26) ccw
  arc A187 (34.3259, 48.9309) -> (34.2541, 48.8591) centre (34.29, 48.895) ccw
  arc A188 (41.275, 50.7492) -> (41.275, 50.8508) centre (41.275, 50.8) ccw
  arc A189 (43.815, 48.2092) -> (43.815, 48.3108) centre (43.815, 48.26) ccw
  line L97 (39.37, 50.165) -> (38.735, 50.8)
  arc A190 (41.8741, 50.1291) -> (41.9459, 50.2009) centre (41.91, 50.165) ccw
  line L98 (41.275, 50.8) -> (40.005, 50.8)
  arc A191 (36.7941, 50.2009) -> (36.8659, 50.1291) centre (36.83, 50.165) ccw
  arc A192 (32.385, 50.8508) -> (32.385, 50.7492) centre (32.385, 50.8) ccw
  arc A193 (38.735, 50.7492) -> (38.735, 50.8508) centre (38.735, 50.8) ccw
  line L99 (44.45, 48.895) -> (43.815, 48.26)
  arc A194 (37.4291, 48.2241) -> (37.5009, 48.2959) centre (37.465, 48.26) ccw
  line L100 (42.545, 48.26) -> (43.815, 48.26)
  line L101 (24.765, 48.26) -> (26.035, 48.26)
  arc A195 (44.4141, 50.1291) -> (44.4859, 50.2009) centre (44.45, 50.165) ccw
  arc A196 (43.7791, 48.2959) -> (43.8509, 48.2241) centre (43.815, 48.26) ccw
  arc A197 (26.035, 48.2092) -> (26.035, 48.3108) centre (26.035, 48.26) ccw
  line L102 (40.005, 48.26) -> (41.275, 48.26)
  line L103 (41.275, 48.26) -> (41.91, 48.895)
  arc A198 (24.765, 48.3108) -> (24.765, 48.2092) centre (24.765, 48.26) ccw
  arc A199 (24.0941, 50.2009) -> (24.1659, 50.1291) centre (24.13, 50.165) ccw
  arc A200 (24.1808, 50.165) -> (24.0792, 50.165) centre (24.13, 50.165) ccw
  arc A201 (25.9991, 48.2959) -> (26.0709, 48.2241) centre (26.035, 48.26) ccw
  line L104 (24.13, 48.895) -> (24.765, 48.26)
  arc A202 (24.8009, 50.7641) -> (24.7291, 50.8359) centre (24.765, 50.8) ccw
  line L105 (39.37, 48.895) -> (40.005, 48.26)
  line L106 (26.035, 50.8) -> (26.67, 50.165)
  arc A203 (39.4059, 48.9309) -> (39.3341, 48.8591) centre (39.37, 48.895) ccw
  line L107 (24.765, 50.8) -> (24.13, 50.165)
  arc A204 (26.7059, 48.8591) -> (26.6341, 48.9309) centre (26.67, 48.895) ccw
  line L108 (26.035, 50.8) -> (24.765, 50.8)
  arc A205 (40.005, 48.3108) -> (40.005, 48.2092) centre (40.005, 48.26) ccw
  arc A206 (41.275, 48.2092) -> (41.275, 48.3108) centre (41.275, 48.26) ccw
  arc A207 (24.765, 50.8508) -> (24.765, 50.7492) centre (24.765, 50.8) ccw
  line L109 (43.815, 50.8) -> (44.45, 50.165)
  arc A208 (24.0792, 48.895) -> (24.1808, 48.895) centre (24.13, 48.895) ccw
  arc A209 (24.1659, 48.9309) -> (24.0941, 48.8591) centre (24.13, 48.895) ccw
  arc A210 (40.0409, 50.7641) -> (39.9691, 50.8359) centre (40.005, 50.8) ccw
  arc A211 (24.7291, 48.2241) -> (24.8009, 48.2959) centre (24.765, 48.26) ccw
  arc A212 (26.035, 50.7492) -> (26.035, 50.8508) centre (26.035, 50.8) ccw
  arc A213 (39.9691, 48.2241) -> (40.0409, 48.2959) centre (40.005, 48.26) ccw
  arc A214 (43.8509, 50.8359) -> (43.7791, 50.7641) centre (43.815, 50.8) ccw
  arc A215 (26.0709, 50.8359) -> (25.9991, 50.7641) centre (26.035, 50.8) ccw
  arc A216 (42.545, 48.3108) -> (42.545, 48.2092) centre (42.545, 48.26) ccw
  arc A217 (41.9459, 48.8591) -> (41.8741, 48.9309) centre (41.91, 48.895) ccw
  arc A218 (26.6341, 50.1291) -> (26.7059, 50.2009) centre (26.67, 50.165) ccw
  arc A219 (44.4859, 48.8591) -> (44.4141, 48.9309) centre (44.45, 48.895) ccw
  line L110 (24.13, 50.165) -> (24.13, 48.895)
  arc A220 (39.3341, 50.2009) -> (39.4059, 50.1291) centre (39.37, 50.165) ccw
  arc A221 (41.2391, 48.2959) -> (41.3109, 48.2241) centre (41.275, 48.26) ccw
  line L111 (26.67, 48.895) -> (26.035, 48.26)
  arc A222 (49.5659, 5.6791) -> (49.4941, 5.7509) centre (49.53, 5.715) ccw
  arc A223 (46.3191, 5.1159) -> (46.3909, 5.0441) centre (46.355, 5.08) ccw
  line L112 (48.895, 5.08) -> (49.53, 5.715)
  arc A224 (46.3909, 7.6559) -> (46.3191, 7.5841) centre (46.355, 7.62) ccw
  arc A225 (47.0259, 5.6791) -> (46.9541, 5.7509) centre (46.99, 5.715) ccw
  arc A226 (37.5009, 7.5841) -> (37.4291, 7.6559) centre (37.465, 7.62) ccw
  line L113 (41.91, 5.715) -> (42.545, 5.08)
  line L114 (40.005, 5.08) -> (39.37, 5.715)
  arc A227 (39.9691, 5.0441) -> (40.0409, 5.1159) centre (40.005, 5.08) ccw
  line L115 (46.99, 6.985) -> (46.355, 7.62)
  line L116 (46.355, 7.62) -> (45.085, 7.62)
  arc A228 (47.625, 5.1308) -> (47.625, 5.0292) centre (47.625, 5.08) ccw
  arc A229 (46.355, 5.0292) -> (46.355, 5.1308) centre (46.355, 5.08) ccw
  arc A230 (44.4859, 5.7509) -> (44.4141, 5.6791) centre (44.45, 5.715) ccw
  line L117 (47.625, 5.08) -> (48.895, 5.08)
  arc A231 (49.4941, 6.9491) -> (49.5659, 7.0209) centre (49.53, 6.985) ccw
  arc A232 (46.9541, 6.9491) -> (47.0259, 7.0209) centre (46.99, 6.985) ccw
  arc A233 (48.8591, 5.1159) -> (48.9309, 5.0441) centre (48.895, 5.08) ccw
  arc A234 (46.355, 7.5692) -> (46.355, 7.6708) centre (46.355, 7.62) ccw
  line L118 (46.355, 5.08) -> (46.99, 5.715)
  line L119 (44.45, 5.715) -> (45.085, 5.08)
  arc A235 (45.0491, 5.0441) -> (45.1209, 5.1159) centre (45.085, 5.08) ccw
  line L120 (46.99, 6.985) -> (47.625, 7.62)
  arc A236 (48.895, 5.0292) -> (48.895, 5.1308) centre (48.895, 5.08) ccw
  line L121 (37.465, 7.62) -> (36.83, 6.985)
  arc A237 (45.085, 7.6708) -> (45.085, 7.5692) centre (45.085, 7.62) ccw
  arc A238 (48.9309, 7.6559) -> (48.8591, 7.5841) centre (48.895, 7.62) ccw
  arc A239 (44.4859, 5.6791) -> (44.4141, 5.7509) centre (44.45, 5.715) ccw
  arc A240 (47.6609, 7.5841) -> (47.5891, 7.6559) centre (47.625, 7.62) ccw
  line L122 (45.085, 5.08) -> (46.355, 5.08)
  arc A241 (42.545, 5.1308) -> (42.545, 5.0292) centre (42.545, 5.08) ccw
  arc A242 (40.005, 5.1308) -> (40.005, 5.0292) centre (40.005, 5.08) ccw
  arc A243 (38.735, 5.0292) -> (38.735, 5.1308) centre (38.735, 5.08) ccw
  line L123 (49.53, 6.985) -> (48.895, 7.62)
  arc A244 (45.085, 5.1308) -> (45.085, 5.0292) centre (45.085, 5.08) ccw
  arc A245 (43.815, 7.5692) -> (43.815, 7.6708) centre (43.815, 7.62) ccw
  arc A246 (47.0259, 5.7509) -> (46.9541, 5.6791) centre (46.99, 5.715) ccw
  arc A247 (39.4059, 5.7509) -> (39.3341, 5.6791) centre (39.37, 5.715) ccw
  line L124 (42.545, 7.62) -> (41.91, 6.985)
  arc A248 (41.3109, 7.6559) -> (41.2391, 7.5841) centre (41.275, 7.62) ccw
  line L125 (41.275, 7.62) -> (40.005, 7.62)
  line L126 (48.895, 7.62) -> (47.625, 7.62)
  arc A249 (38.735, 7.5692) -> (38.735, 7.6708) centre (38.735, 7.62) ccw
  arc A250 (38.7709, 7.6559) -> (38.6991, 7.5841) centre (38.735, 7.62) ccw
  arc A251 (41.275, 5.0292) -> (41.275, 5.1308) centre (41.275, 5.08) ccw
  line L127 (37.465, 5.08) -> (38.735, 5.08)
  arc A252 (36.8659, 5.7509) -> (36.7941, 5.6791) centre (36.83, 5.715) ccw
  arc A253 (39.3341, 7.0209) -> (39.4059, 6.9491) centre (39.37, 6.985) ccw
  arc A254 (41.9459, 5.7509) -> (41.8741, 5.6791) centre (41.91, 5.715) ccw
  line L128 (38.735, 5.08) -> (39.37, 5.715)
  arc A255 (45.1209, 7.5841) -> (45.0491, 7.6559) centre (45.085, 7.62) ccw
  arc A256 (42.5091, 5.0441) -> (42.5809, 5.1159) centre (42.545, 5.08) ccw
  arc A257 (43.8509, 7.6559) -> (43.7791, 7.5841) centre (43.815, 7.62) ccw
  line L129 (43.815, 7.62) -> (42.545, 7.62)
  arc A258 (43.7791, 5.1159) -> (43.8509, 5.0441) centre (43.815, 5.08) ccw
  arc A259 (48.895, 7.5692) -> (48.895, 7.6708) centre (48.895, 7.62) ccw
  arc A260 (37.465, 5.1308) -> (37.465, 5.0292) centre (37.465, 5.08) ccw
  arc A261 (41.9459, 5.6791) -> (41.8741, 5.7509) centre (41.91, 5.715) ccw
  line L130 (38.735, 7.62) -> (37.465, 7.62)
  arc A262 (37.4291, 5.0441) -> (37.5009, 5.1159) centre (37.465, 5.08) ccw
  arc A263 (34.2541, 6.9491) -> (34.3259, 7.0209) centre (34.29, 6.985) ccw
  arc A264 (36.1591, 5.1159) -> (36.2309, 5.0441) centre (36.195, 5.08) ccw
  line L131 (47.625, 5.08) -> (46.99, 5.715)
  arc A265 (42.545, 7.6708) -> (42.545, 7.5692) centre (42.545, 7.62) ccw
  arc A266 (41.2391, 5.1159) -> (41.3109, 5.0441) centre (41.275, 5.08) ccw
  line L132 (42.545, 5.08) -> (43.815, 5.08)
  arc A267 (41.8741, 7.0209) -> (41.9459, 6.9491) centre (41.91, 6.985) ccw
  arc A268 (34.9609, 7.5841) -> (34.8891, 7.6559) centre (34.925, 7.62) ccw
  line L133 (31.75, 5.715) -> (31.75, 6.985)
  arc A269 (31.7859, 5.7509) -> (31.7141, 5.6791) centre (31.75, 5.715) ccw
  arc A270 (36.8659, 5.6791) -> (36.7941, 5.7509) centre (36.83, 5.715) ccw
  arc A271 (46.9541, 7.0209) -> (47.0259, 6.9491) centre (46.99, 6.985) ccw
  arc A272 (47.625, 7.6708) -> (47.625, 7.5692) centre (47.625, 7.62) ccw
  arc A273 (39.4059, 5.6791) -> (39.3341, 5.7509) centre (39.37, 5.715) ccw
  arc A274 (38.6991, 5.1159) -> (38.7709, 5.0441) centre (38.735, 5.08) ccw
  line L134 (39.37, 6.985) -> (38.735, 7.62)
  arc A275 (37.465, 7.6708) -> (37.465, 7.5692) centre (37.465, 7.62) ccw
  arc A276 (34.8891, 5.0441) -> (34.9609, 5.1159) centre (34.925, 5.08) ccw
  arc A277 (36.7941, 7.0209) -> (36.8659, 6.9491) centre (36.83, 6.985) ccw
  line L135 (41.91, 6.985) -> (41.275, 7.62)
  arc A278 (36.2309, 7.6559) -> (36.1591, 7.5841) centre (36.195, 7.62) ccw
  arc A279 (31.8008, 6.985) -> (31.6992, 6.985) centre (31.75, 6.985) ccw
  line L136 (45.085, 7.62) -> (44.45, 6.985)
  line L137 (36.83, 5.715) -> (37.465, 5.08)
  line L138 (43.815, 5.08) -> (44.45, 5.715)
  line L139 (41.275, 5.08) -> (41.91, 5.715)
  arc A280 (44.4141, 6.9491) -> (44.4859, 7.0209) centre (44.45, 6.985) ccw
  line L140 (40.005, 5.08) -> (41.275, 5.08)
  arc A281 (42.5809, 7.5841) -> (42.5091, 7.6559) centre (42.545, 7.62) ccw
  line L141 (34.925, 7.62) -> (34.29, 6.985)
  line L142 (44.45, 6.985) -> (43.815, 7.62)
  line L143 (39.37, 6.985) -> (40.005, 7.62)
  arc A282 (32.3491, 5.0441) -> (32.4209, 5.1159) centre (32.385, 5.08) ccw
  arc A283 (34.3259, 5.7509) -> (34.2541, 5.6791) centre (34.29, 5.715) ccw
  arc A284 (32.385, 5.1308) -> (32.385, 5.0292) centre (32.385, 5.08) ccw
  arc A285 (32.4209, 7.5841) -> (32.3491, 7.6559) centre (32.385, 7.62) ccw
  arc A286 (39.3341, 6.9491) -> (39.4059, 7.0209) centre (39.37, 6.985) ccw
  arc A287 (43.815, 5.0292) -> (43.815, 5.1308) centre (43.815, 5.08) ccw
  arc A288 (41.8741, 6.9491) -> (41.9459, 7.0209) centre (41.91, 6.985) ccw
  arc A289 (40.0409, 7.5841) -> (39.9691, 7.6559) centre (40.005, 7.62) ccw
  arc A290 (47.5891, 5.0441) -> (47.6609, 5.1159) centre (47.625, 5.08) ccw
  arc A291 (44.4141, 7.0209) -> (44.4859, 6.9491) centre (44.45, 6.985) ccw
  arc A292 (64.8059, 5.6791) -> (64.7341, 5.7509) centre (64.77, 5.715) ccw
  line L144 (66.675, 5.08) -> (67.31, 5.715)
  arc A293 (61.595, 5.0292) -> (61.595, 5.1308) centre (61.595, 5.08) ccw
  arc A294 (64.7341, 6.9491) -> (64.8059, 7.0209) centre (64.77, 6.985) ccw
  arc A295 (34.3259, 5.6791) -> (34.2541, 5.7509) centre (34.29, 5.715) ccw
  arc A296 (36.195, 5.0292) -> (36.195, 5.1308) centre (36.195, 5.08) ccw
  arc A297 (64.0991, 5.1159) -> (64.1709, 5.0441) centre (64.135, 5.08) ccw
  arc A298 (66.7109, 7.6559) -> (66.6391, 7.5841) centre (66.675, 7.62) ccw
  arc A299 (34.925, 5.1308) -> (34.925, 5.0292) centre (34.925, 5.08) ccw
  line L145 (64.77, 6.985) -> (64.135, 7.62)
  line L146 (36.83, 6.985) -> (36.195, 7.62)
  arc A300 (64.1709, 7.6559) -> (64.0991, 7.5841) centre (64.135, 7.62) ccw
  arc A301 (36.195, 7.5692) -> (36.195, 7.6708) centre (36.195, 7.62) ccw
  arc A302 (33.6191, 5.1159) -> (33.6909, 5.0441) centre (33.655, 5.08) ccw
  arc A303 (66.6391, 5.1159) -> (66.7109, 5.0441) centre (66.675, 5.08) ccw
  line L147 (34.925, 5.08) -> (36.195, 5.08)
  arc A304 (34.2541, 7.0209) -> (34.3259, 6.9491) centre (34.29, 6.985) ccw
  line L148 (62.865, 5.08) -> (64.135, 5.08)
  arc A305 (32.385, 7.6708) -> (32.385, 7.5692) centre (32.385, 7.62) ccw
  arc A306 (67.2741, 6.9491) -> (67.3459, 7.0209) centre (67.31, 6.985) ccw
  arc A307 (33.655, 7.5692) -> (33.655, 7.6708) centre (33.655, 7.62) ccw
  arc A308 (40.005, 7.6708) -> (40.005, 7.5692) centre (40.005, 7.62) ccw
  arc A309 (36.7941, 6.9491) -> (36.8659, 7.0209) centre (36.83, 6.985) ccw
  line L149 (62.23, 5.715) -> (62.865, 5.08)
  arc A310 (62.2659, 5.7509) -> (62.1941, 5.6791) centre (62.23, 5.715) ccw
  line L150 (55.245, 5.08) -> (56.515, 5.08)
  arc A311 (67.3459, 5.6791) -> (67.2741, 5.7509) centre (67.31, 5.715) ccw
  arc A312 (62.865, 5.1308) -> (62.865, 5.0292) centre (62.865, 5.08) ccw
  line L151 (54.61, 5.715) -> (55.245, 5.08)
  line L152 (56.515, 5.08) -> (57.15, 5.715)
  arc A313 (65.4409, 7.5841) -> (65.3691, 7.6559) centre (65.405, 7.62) ccw
  arc A314 (59.055, 5.0292) -> (59.055, 5.1308) centre (59.055, 5.08) ccw
  line L153 (34.29, 6.985) -> (33.655, 7.62)
  arc A315 (33.6909, 7.6559) -> (33.6191, 7.5841) centre (33.655, 7.62) ccw
  line L154 (31.75, 6.985) -> (32.385, 7.62)
  line L155 (59.69, 5.715) -> (60.325, 5.08)
  arc A316 (57.1859, 5.6791) -> (57.1141, 5.7509) centre (57.15, 5.715) ccw
  arc A317 (59.0191, 5.1159) -> (59.0909, 5.0441) centre (59.055, 5.08) ccw
  arc A318 (56.5509, 7.6559) -> (56.4791, 7.5841) centre (56.515, 7.62) ccw
  line L156 (32.385, 5.08) -> (33.655, 5.08)
  arc A319 (54.6459, 5.7509) -> (54.5741, 5.6791) centre (54.61, 5.715) ccw
  line L157 (36.195, 5.08) -> (36.83, 5.715)
  line L158 (33.655, 5.08) -> (34.29, 5.715)
  line L159 (32.385, 5.08) -> (31.75, 5.715)
  line L160 (57.15, 6.985) -> (56.515, 7.62)
  arc A320 (55.245, 5.1308) -> (55.245, 5.0292) centre (55.245, 5.08) ccw
  arc A321 (34.925, 7.6708) -> (34.925, 7.5692) centre (34.925, 7.62) ccw
  arc A322 (31.7141, 7.0209) -> (31.7859, 6.9491) centre (31.75, 6.985) ccw
  line L161 (64.135, 5.08) -> (64.77, 5.715)
  arc A323 (41.275, 7.5692) -> (41.275, 7.6708) centre (41.275, 7.62) ccw
  arc A324 (65.405, 5.1308) -> (65.405, 5.0292) centre (65.405, 5.08) ccw
  line L162 (67.31, 6.985) -> (66.675, 7.62)
  arc A325 (64.135, 5.0292) -> (64.135, 5.1308) centre (64.135, 5.08) ccw
  arc A326 (33.655, 5.0292) -> (33.655, 5.1308) centre (33.655, 5.08) ccw
  line L163 (59.055, 5.08) -> (59.69, 5.715)
  line L164 (65.405, 5.08) -> (66.675, 5.08)